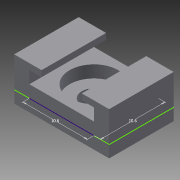
# Autodesk Inventor part: MicroUSBClip
Saved by Autodesk Inventor 2015 (Build 190159000, 159)
## iProperties
Created: 2015-05-12
Part Number: MicroUSBClip
Material: Generic
Document SubType Name: Modeling
Designer: Quinn
Density: 1 g/cm^3
Appearance: Default
Author: Quinn
Autodesk Inventor part; units mm, degrees
ref_plane "YZ Plane" through (0, 0, 0) normal (1, 0, 0) x (0, 1, 0)
ref_plane "XZ Plane" through (0, 0, 0) normal (0, 1, 0) x (-1, 0, 0)
ref_plane "XY Plane" through (0, 0, 0) normal (0, 0, 1) x (1, 0, 0)
sketch "Sketch1" plane through (0, 0, 0) normal (0, 1, 0) x (-1, 0, 0)
  line L0 (5.3, -5.3) -> (-5.3, -5.3)
  line L1 (-5.3, -5.3) -> (-5.3, 5.3)
  line L2 (-5.3, 5.3) -> (5.3, 5.3)
  line L3 (5.3, 5.3) -> (5.3, -5.3)
  line L4 (7.8, -5.3) -> (7.8, 5.3)
  line L5 (-7.8, 5.3) -> (-7.8, -5.3)
  line L6 (5.3, -5.3) -> (7.8, -5.3)
  line L7 (-5.3, -5.3) -> (-7.8, -5.3)
  line L8 (-5.3, 5.3) -> (-7.8, 5.3)
  line L9 (5.3, 5.3) -> (7.8, 5.3)
  point P0 (0, 0)
  point P1 (-5.3, 0)
  point P2 (0, -5.3)
  dimension "d0" = 10.6
  dimension "d1" = 10.6
  constraints: 20 end point, 4 parallel, 2 midpoint, 2 perpendicular, 2 point on line, 1 horizontal, 1 horizontal alignment, 1 vertical alignment
  measures "d0" distance of L1.end L2.end
  measures "d1" distance of L0.end L1.end
extrude "Extrusion1" add sketch "Sketch1" along normal blind 2
extrude "Extrusion2" add sketch "Sketch1" along normal blind 5 contours L3 L9 L4 L6 | L7 L5 L8 L1
sketch "Sketch2" plane through (-5.3, 2, -5.3) normal (1, 0, 0) x (0, 0, -1)
  line L0 (0, 0) -> (-10.6, 0) projected
  line L1 (0, 0) -> (0, 3) projected
  line L2 (-10.6, 3) -> (0, 3) projected
  line L3 (-10.6, 0) -> (-10.6, 3) projected
  line L4 (-10.6, 3) -> (0, 3)
  line L5 (0, 3) -> (0, 2)
  line L6 (0, 2) -> (-10.6, 2)
  line L7 (-10.6, 2) -> (-10.6, 3)
  point P0 (-5.3, -2)
  dimension "d7" = 1
  constraints: 8 end point, 2 parallel, 1 horizontal, 1 perpendicular, 1 point on line
  measures "d7" distance of L4.end L5.end
extrude "Extrusion3" add sketch "Sketch2" along normal blind 2 contours L6 L3 L2 L1
mirror "Mirror1" about plane through (0, 0, 0) normal (1, 0, 0) of "Extrusion3"
move faces "Move1" translate (0, -2, 0) faces at (-2.6, 0, 1.7667)
sketch "Sketch3" plane through (-7.8, -2, -5.3) normal (0, -1, 0) x (1, 0, 0)
  line L0 (15.6, 0) -> (0, 0) projected
  line L1 (15.6, 10.6) -> (15.6, 0) projected
  line L2 (0, 10.6) -> (15.6, 10.6) projected
  line L3 (0, 0) -> (0, 10.6) projected
  line L4 (7.8, 10.6) -> (7.8, 0)
  circle A0 centre (7.8, 5.3) radius 2
  dimension "d13" = 4
  constraints: 2 end point, 2 midpoint, 1 centre point, 1 coincident
  measures "d13" diameter of A0
extrude "Extrusion4" cut sketch "Sketch3" against normal through all contours A0 L4 | L4 A0
sketch "Sketch4" plane through (0, 2, 0) normal (0, 1, 0) x (1, 0, 0)
  circle A0 centre (0, 0) radius 2 projected
  line L0 (-5.3, 5.3) -> (-5.3, -5.3) projected
  line L1 (-5.3, -5.3) -> (5.3, -5.3) projected
  line L2 (5.3, -5.3) -> (5.3, 5.3) projected
  line L3 (5.3, 5.3) -> (-5.3, 5.3) projected
  circle A1 centre (0, 0) radius 4
  dimension "d16" = 2
  constraints: 1 centre point
  measures "d16" radial gap between concentric circles of A0 A1
extrude "Extrusion5" cut sketch "Sketch4" against normal blind 2 contours A1
body "Solid1"
